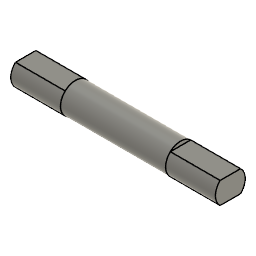
Axis (Autodesk Fusion 360 design; units mm, degrees)
part number: 2026-01-03-02-12-30-808
Autodesk Fusion 360 part; units mm, degrees
sketch "Center" plane through (0, 0, 0) normal (1, 0, 0) x (0, 1, 0)
  circle A0 centre (0, 0) radius 2.7
  dimension "d1" = 5.4
  constraint coincident A0.centre origin
  measures "d1" diameter of A0
extrude "Center width" add sketch "Center" along normal blind 19 makes body 1
sketch "Axis" plane through (19, 0, 0) normal (1, 0, 0) x (0, 1, 0)
  circle A0 centre (0, 0) radius 2.7
  line L0 (-1.85, 1.9666) -> (1.85, 1.9666)
  line L1 (1.85, -1.9666) -> (-1.85, -1.9666)
  arc A1 (-1.85, 1.9666) -> (-1.85, -1.9666) centre (0, 0) ccw
  arc A2 (1.85, -1.9666) -> (1.85, 1.9666) centre (0, 0) ccw
  dimension "d4" = 5.4
  dimension "d5" = 3.7
  constraint coincident A0.centre A1.centre
  constraint horizontal L0
  constraint parallel L0 L1
  constraint coincident A0 L0.start
  constraint concentric A1 A2
  measures "d4" diameter of A1
  measures "d5" distance of L0.start L0.end
extrude "Axis width" add sketch "Axis" along normal blind 9 separate body contours A0 L0 L1 A1 A2 makes body 2
ref_plane "WorkPlane1" through (9.5, 0, 0) normal (1, 0, 0) x (0, 1, 0)
mirror "Axis mirror" about plane through (9.5, 0, 0) normal (1, 0, 0) of "Axis width" makes body 3
equation "d8 = ( 19 / 2 ) * 1 mm"
named bodies: "Center", "Axis part 1", "Axis part 2"
